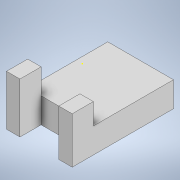
# Autodesk Inventor part: 공부용
Saved by Autodesk Inventor 2022 (Build 260153000, 153)
## iProperties
Created: 2021-08-05
Part Number: 공부용
Material: 일반
Document SubType Name: Modeling
Designer: user
Density: 1 g/cm^3
Appearance: 기본값
Author: user
Autodesk Inventor part; units mm, degrees
ref_plane "YZ Plane" through (0, 0, 0) normal (1, 0, 0) x (0, 1, 0)
ref_plane "XZ Plane" through (0, 0, 0) normal (0, 1, 0) x (-1, 0, 0)
ref_plane "XY Plane" through (0, 0, 0) normal (0, 0, 1) x (1, 0, 0)
sketch "스케치2" plane through (0, 0, 0) normal (0, 1, 0) x (-1, 0, 0)
  line L0 (12.4336, 17.7711) -> (-13.7162, 17.7711)
  line L1 (-13.7162, 17.7711) -> (-13.7162, -22.5294)
  line L2 (-13.7162, -22.5294) -> (12.4336, -22.5294)
  line L3 (12.4336, -22.5294) -> (12.4336, 17.7711)
  point P0 (0, 0)
  constraints: 8 end point, 2 parallel, 1 horizontal, 1 perpendicular
extrude "돌출1" add sketch "스케치2" along normal blind 10
sketch "스케치3" plane through (0, 10, 0) normal (0, 1, 0) x (1, 0, 0)
  line L0 (-12.4336, 22.5294) -> (-12.4336, -17.7711) projected
  line L1 (-12.4336, -17.7711) -> (-7.0874, -17.7711)
  line L2 (-7.0874, -17.7711) -> (-7.0874, -9.3549)
  line L3 (-7.0874, -9.3549) -> (-12.4336, -9.3549)
  line L4 (-12.4336, -9.3549) -> (-12.4336, -17.7711)
  point P0 (0, 0)
  constraints: 8 end point, 2 parallel, 1 horizontal, 1 perpendicular
extrude "돌출2" add sketch "스케치3" along normal blind 10
sketch "스케치4" plane through (0, 10, 0) normal (0, 1, 0) x (1, 0, 0)
  line L0 (-12.4336, -17.7711) -> (13.7162, -17.7711) projected
  line L1 (13.7162, -17.7711) -> (8.3702, -17.7711)
  line L2 (8.3702, -17.7711) -> (8.3702, -9.3551)
  line L3 (8.3702, -9.3551) -> (13.7162, -9.3551)
  line L4 (13.7162, -9.3551) -> (13.7162, -17.7711)
  point P0 (0, 0)
  dimension "d4" = 5.346
  dimension "d5" = 8.416
  constraints: 8 end point, 2 parallel, 1 horizontal, 1 perpendicular
  measures "d4" distance of L2.end L3.end
  measures "d5" distance of L1.end L2.end
extrude "돌출3" add sketch "스케치4" along normal blind 8.416
sketch "스케치5" plane through (-12.4336, 0, 17.7711) normal (0, 0, 1) x (1, 0, 0)
  line L0 (5.3461, 10) -> (20.8038, 10) projected
  line L1 (0, 0) -> (26.1498, 0) projected
  line L2 (5.3461, 10) -> (20.8037, 10)
  line L3 (20.8037, 10) -> (20.8037, 0)
  line L4 (20.8037, 0) -> (5.3461, 0)
  line L5 (5.3461, 0) -> (5.3461, 10)
  point P0 (12.4336, 0)
  dimension "d8" = 26.1498
  constraints: 8 end point, 2 parallel, 1 horizontal, 1 perpendicular, 1 point on line
  measures "d8" distance of L1.start L1.end
sketch "스케치6" plane through (0, 20, 0) normal (0, 1, 0) x (1, 0, 0)
  point P0 (0, 0)
extrude "돌출4" cut sketch "스케치5" against normal blind 8.416
equation "\"d6\" = d5"
